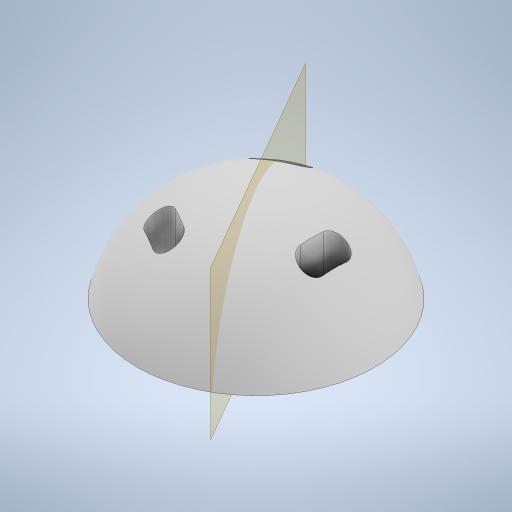
# Autodesk Inventor part: hemisphere_1
Saved by Autodesk Inventor 2024.2 (Build 282272000, 272)
## iProperties
Created: 2024-06-17
Part Number: hemisphere_1
Material: Ogólny
Document SubType Name: Modeling
Designer: Konrad
Density: 1 g/cm^3
Appearance: Domyślna
Author: Konrad
Autodesk Inventor part; units mm, degrees
ref_plane "YZ Plane" through (0, 0, 0) normal (1, 0, 0) x (0, 1, 0)
ref_plane "XZ Plane" through (0, 0, 0) normal (0, 1, 0) x (-1, 0, 0)
ref_plane "XY Plane" through (0, 0, 0) normal (0, 0, 1) x (1, 0, 0)
sketch "Szkic1" plane through (0, 0, 0) normal (0, 1, 0) x (-1, 0, 0)
  circle A0 centre (0, 0) radius 19.62 construction
  line L0 (0, 0) -> (-19.62, 0) construction
  circle A1 centre (0, 0) radius 22.5 construction
  circle A2 centre (-19.3219, 3.407) radius 1.75
  circle A3 centre (-19.3219, -3.407) radius 1.75
  circle A4 centre (6.7104, 18.4368) radius 1.75
  circle A5 centre (12.6115, 15.0298) radius 1.75
  circle A6 centre (12.6115, -15.0298) radius 1.75
  circle A7 centre (6.7104, -18.4368) radius 1.75
  circle A8 centre (0, 0) radius 35
  circle A9 centre (-19.3219, 3.407) radius 3.25
  circle A10 centre (-19.3219, -3.407) radius 3.25
  circle A11 centre (6.7104, -18.4368) radius 3.25
  circle A12 centre (12.6115, -15.0298) radius 3.25
  circle A13 centre (12.6115, 15.0298) radius 3.25
  circle A14 centre (6.7104, 18.4368) radius 3.25
  line L1 (14.2365, 17.8444) -> (8.3354, 21.2514)
  line L2 (10.9865, 12.2152) -> (5.0854, 15.6222)
  line L3 (-16.0719, 3.407) -> (-16.0719, -3.407)
  line L4 (14.2365, -17.8444) -> (8.3354, -21.2514)
  line L5 (10.9865, -12.2152) -> (5.0854, -15.6222)
  line L6 (-22.5719, -3.407) -> (-22.5719, 3.407)
  dimension "d0" = 39.24
  dimension "d1" = 3.5
  dimension "d2" = 20
  dimension "d5" = 360
  dimension "d7" = 45
  dimension "d8" = 70
  dimension "d12" = 6.5
  dimension "d15" = 360
  constraints: 15 centre point, 15 point on circle, 14 end point, 12 tangent, 5 coincident, 2 equal radius, 1 horizontal, 1 symmetric about line, 26 other
  measures "d0" diameter of A0
  measures "d1" diameter of A2
  measures "d7" diameter of A1
  measures "d8" diameter of A8
  measures "d12" diameter of A9
sketch "Szkic3" plane through (0, 0, 0) normal (0, 0, 1) x (1, 0, 0)
  arc A0 (0, 35) -> (-35, 0) centre (0, 0) ccw
  line L0 (0, 35) -> (0, 0)
  line L1 (0, 0) -> (-35, 0)
  line L2 (0, -8.4497) -> (0, 50.6985) projected
  dimension "d19" = 35
  constraints: 4 end point, 2 point on circle, 1 centre point, 1 coincident, 1 perpendicular, 1 vertical
  measures "d19" radius of A0
revolve "Obrót1" add sketch "Szkic3" angle 360 about axis through (0, -10, 0) along (0, 1, 0)
extrude "Wyciągnięcie proste1" cut sketch "Szkic1" along normal through all contours A2 | A3 | A4 | A5 | A6 | A7 | A9 | L3 A10 L6 A9 | A10 | A11 | A11 L5 A12 L4 | A12 | A13 | A13 L2 A14 L1 | A14
extrude "Wyciągnięcie proste2" add sketch "Szkic1" along normal blind 17.85 contours A9 | L3 A10 L6 A9 | A10 | A11 | A11 L5 A12 L4 | A12 | A13 | A13 L2 A14 L1 | A14
extrude "Wyciągnięcie proste3" cut sketch "Szkic1" along normal blind 7.85 contours A2 | A3 | A4 | A5 | A6 | A7 | A8 | A9 | L3 A10 L6 A9 | A10 | A11 | A11 L5 A12 L4 | A12 | A13 | A13 L2 A14 L1 | A14
ref_plane "Płaszczyzna konstrukcyjna2" through (-11.286, 17.85, -19.5479) normal (-0.866, 0, 0.5) x (0.5, 0, 0.866)
